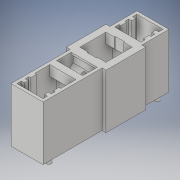
# Autodesk Inventor part: Colorimeter
Saved by Autodesk Inventor 2019 (Build 230136000, 136)
## iProperties
Created: 2019-03-27
Part Number: Colorimeter
Material: Generic
Document SubType Name: Modeling
Designer: Hansen
Density: 1 g/cm^3
Appearance: Default
Author: Hansen
Autodesk Inventor part; units mm, degrees
ref_plane "YZ Plane" through (0, 0, 0) normal (1, 0, 0) x (0, 1, 0)
ref_plane "XZ Plane" through (0, 0, 0) normal (0, 1, 0) x (-1, 0, 0)
ref_plane "XY Plane" through (0, 0, 0) normal (0, 0, 1) x (1, 0, 0)
sketch "BasePlateSketch" plane through (0, 0, 0) normal (0, 1, 0) x (-1, 0, 0)
  line L0 (-8.25, 32.5) -> (8.25, 32.5)
  line L1 (8.25, 32.5) -> (8.25, -32.5)
  line L2 (8.25, -32.5) -> (-8.25, -32.5)
  line L3 (-8.25, -32.5) -> (-8.25, 32.5)
  line L4 (-8.25, 32.5) -> (8.25, -32.5) construction
  line L5 (8.25, 32.5) -> (-8.25, -32.5) construction
  circle A0 centre (0, 28) radius 1.35
  circle A1 centre (0, -28) radius 1.35
  line L6 (-5.85, -25.25) -> (5.85, -25.25)
  line L7 (5.85, -25.25) -> (5.85, -21.75)
  line L8 (5.85, -21.75) -> (-5.85, -21.75)
  line L9 (-5.85, -21.75) -> (-5.85, -25.25)
  line L10 (-5.85, -25.25) -> (5.85, -21.75) construction
  line L11 (5.85, -25.25) -> (-5.85, -21.75) construction
  line L12 (-5.85, 25.25) -> (5.85, 25.25)
  line L13 (5.85, 25.25) -> (5.85, 21.75)
  line L14 (5.85, 21.75) -> (-5.85, 21.75)
  line L15 (-5.85, 21.75) -> (-5.85, 25.25)
  line L16 (-5.85, 25.25) -> (5.85, 21.75) construction
  line L17 (5.85, 25.25) -> (-5.85, 21.75) construction
  line L18 (4.375, 7) -> (-4.375, 7)
  line L19 (-4.375, 7) -> (-4.375, 2)
  line L20 (-4.375, 2) -> (4.375, 2)
  line L21 (4.375, 2) -> (4.375, 7)
  line L22 (4.375, 7) -> (-4.375, 2) construction
  line L23 (-4.375, 7) -> (4.375, 2) construction
  point P0 (0, 0)
  point P1 (0, 0)
  point P2 (0, 0)
  point P3 (0, -23.5)
  point P4 (0, -23.5)
  point P5 (0, 23.5)
  point P6 (0, 23.5)
  point P7 (0, 4.5)
  point P8 (0, 4.5)
  dimension "d0" = 16.5
  dimension "d1" = 65
  dimension "d2" = 4.5
  dimension "d3" = 2.7
  dimension "d4" = 4.5
  dimension "d21" = 11.7
  dimension "d22" = 3.5
  dimension "d23" = 9
  dimension "d24" = 9
  dimension "d25" = 5
  dimension "d26" = 8.75
  dimension "d27" = 25.5
  constraints: 48 end point, 13 midpoint, 8 parallel, 5 vertical alignment, 4 horizontal, 4 perpendicular, 2 centre point, 2 equal length, 1 equal radius
  measures "d0" distance of L1.end L2.end
  measures "d1" distance of L0.end L1.end
  measures "d2" distance from line of L2 A1.centre
  measures "d3" diameter of A1
  measures "d4" distance from line of L0 A0.centre
  measures "d21" distance of L6.start L6.end
  measures "d22" distance of L6.end L7.end
  measures "d23" distance from line of L2 point (0, -23.5)
  measures "d24" distance from line of point (0, 23.5) L0
  measures "d25" distance of L18.end L19.end
  measures "d26" distance of L18.start L18.end
  measures "d27" distance between parallel lines of L0 L18
extrude "BasePlate" add sketch "BasePlateSketch" along normal blind 3
sketch "SeparationsSketch" plane through (8.25, 0, 32.5) normal (1, 0, 0) x (0, 0, -1)
  line L0 (0, 3) -> (65, 3) projected
  line L1 (47.5, 3) -> (51, 3)
  line L2 (47.5, 3) -> (47.5, 5)
  line L3 (47.5, 5) -> (51, 8.5)
  line L4 (51, 8.5) -> (51, 19.25)
  line L5 (51, 19.25) -> (47.5, 22.75)
  line L6 (47.5, 22.75) -> (47.5, 28)
  line L7 (47.5, 28) -> (51, 28)
  line L8 (51, 28) -> (51, 22.75)
  line L9 (51, 22.75) -> (54.5, 19.25)
  line L10 (54.5, 19.25) -> (54.5, 8.5)
  line L11 (54.5, 8.5) -> (51, 5)
  line L12 (51, 5) -> (51, 3)
  line L13 (30.5, 3) -> (34, 3)
  line L14 (34, 3) -> (34, 13)
  line L15 (34, 13) -> (30.5, 16.5)
  line L16 (30.5, 16.5) -> (30.5, 19.25)
  line L17 (30.5, 19.25) -> (34, 22.75)
  line L18 (34, 22.75) -> (34, 28)
  line L19 (34, 28) -> (30.5, 28)
  line L20 (30.5, 28) -> (30.5, 22.75)
  line L21 (30.5, 22.75) -> (27, 19.25)
  line L22 (27, 19.25) -> (27, 16.5)
  line L23 (27, 16.5) -> (30.5, 13)
  line L24 (30.5, 13) -> (30.5, 3)
  line L25 (25.5, 0) -> (25.5, 3) projected
  line L26 (25.5, 3) -> (22, 3)
  line L27 (65, 3) -> (0, 3) projected
  line L28 (25.5, 3) -> (25.5, 19.25)
  line L29 (25.5, 19.25) -> (22, 22.75)
  line L30 (22, 22.75) -> (22, 28)
  line L31 (22, 28) -> (18.5, 28)
  line L32 (22, 3) -> (22, 19.25)
  line L33 (22, 19.25) -> (18.5, 22.75)
  line L34 (18.5, 22.75) -> (18.5, 28)
  point P0 (32.5, 0)
  point P1 (52.75, 21)
  point P2 (49.25, 21)
  point P3 (52.75, 6.75)
  point P4 (49.25, 6.75)
  point P5 (32.25, 21)
  point P6 (28.75, 21)
  point P7 (32.25, 14.75)
  point P8 (28.75, 14.75)
  point P9 (23.75, 21)
  point P10 (20.25, 21)
  dimension "d7" = 3.5
  dimension "d8" = 3.5
  dimension "d9" = 14
  dimension "d10" = 18
  dimension "d11" = 25
  dimension "d13" = 2
  dimension "d14" = 135
  dimension "d16" = 3.5
  dimension "d18" = 13.5
  dimension "d19" = 10
  dimension "d20" = 135
  dimension "d28" = 135
  constraints: 64 end point, 12 parallel, 11 point on line, 10 midpoint, 9 horizontal alignment, 8 perpendicular, 4 vertical, 3 collinear, 3 vertical alignment
  measures "d7" distance between parallel lines of L8 L6
  measures "d8" distance between parallel lines of L10 L4
  measures "d9" distance of L0.end L1.end
  measures "d10" distance from line of L1 point (52.75, 21)
  measures "d11" distance between parallel lines of L1 L7
  measures "d13" distance of L1.start L2.end
  measures "d14" angle of L4 L5
  measures "d16" distance between parallel lines of L16 L22
  measures "d18" distance between parallel lines of L6 L18
  measures "d19" distance of L13.end L14.end
  measures "d20" angle of L16 L17
  measures "d28" angle of L32 L33
extrude "Separations" add sketch "SeparationsSketch" against normal blind 16.5
sketch "Aperture1Sketch" plane through (8.25, 22.75, 14) normal (0, 0, 1) x (1, 0, 0)
  circle A0 centre (-8.25, -1.75) radius 1.5
  line L0 (-16.5, -19.75) -> (0, -19.75) projected
  line L1 (0, -22.75) -> (-16.5, -22.75) projected
  point P0 (-8.25, -22.75)
  point P1 (-8.25, -22.75)
  dimension "d31" = 3
  dimension "d32" = 18
  constraints: 1 centre point, 1 midpoint, 1 vertical alignment
  measures "d31" diameter of A0
  measures "d32" distance from line of L0 A0.centre
extrude "Aperture1" cut sketch "Aperture1Sketch" against normal up to surface (8.5 mm away)
sketch "Aperture2Sketch" plane through (8.25, 16.5, 5.5) normal (0, 0, 1) x (1, 0, 0)
  circle A0 centre (-8.25, 4.5) radius 1.5 projected
  circle A1 centre (-8.25, 4.5) radius 1.375
  point P0 (-8.25, -16.5)
  dimension "d35" = 2.75
  constraints: 1 centre point, 1 coincident
  measures "d35" diameter of A1
extrude "Aperture2" cut sketch "Aperture2Sketch" against normal up to surface (20.5 mm away) contours A1
sketch "Aperture3Sketch" plane through (8.25, 8.5, -22) normal (0, 0, -1) x (-1, 0, 0)
  circle A0 centre (8.25, 12.5) radius 1.375 projected
  circle A1 centre (8.25, 12.5) radius 1
  point P0 (8.25, -8.5)
  point P1 (7.989, 11.65)
  point P2 (7.989, 14.35)
  dimension "d38" = 2
  constraints: 1 centre point, 1 coincident, 1 other
  measures "d38" diameter of A1
extrude "Aperture3" cut sketch "Aperture3Sketch" against normal up to surface (20.5 mm away) contours A1
sketch "ApertureRefSketch" plane through (8.25, 3, 10.5) normal (0, 0, 1) x (1, 0, 0)
  line L0 (-16.5, 0) -> (0, 0) projected
  line L1 (-9.75, 7) -> (-6.75, 7)
  line L2 (-6.75, 7) -> (-6.75, 0)
  line L3 (-6.75, 0) -> (-9.75, 0)
  line L4 (-9.75, 0) -> (-9.75, 7)
  line L5 (-9.75, 7) -> (-6.75, 0) construction
  line L6 (-6.75, 7) -> (-9.75, 0) construction
  line L7 (0, -3) -> (-16.5, -3) projected
  point P0 (-8.25, -3)
  point P1 (-8.25, 3.5)
  point P2 (-8.25, 3.5)
  point P3 (-8.25, -3)
  dimension "d41" = 7
  dimension "d42" = 3
  constraints: 12 end point, 4 midpoint, 2 parallel, 1 horizontal, 1 perpendicular, 1 point on line, 1 vertical alignment
  measures "d41" distance of L3.end L1.start
  measures "d42" distance of L1.start L1.end
extrude "ApertureRef" cut sketch "ApertureRefSketch" against normal up to next
chamfer "ApertureRefChamfer" distance 3 angle 45 1 edges at (0, 10, 10.5)
sketch "OverlapSketch" plane through (8.25, 28, -15) normal (0, 1, 0) x (1, 0, 0)
  line L0 (0, 0) -> (-16.5, 0) projected
  line L1 (0, 17.5) -> (0, -47.5) projected
  line L2 (-16.5, 0) -> (0, 0)
  line L3 (0, 0) -> (0, 4.5)
  line L4 (0, 4.5) -> (-16.5, 4.5)
  line L5 (-16.5, 4.5) -> (-16.5, 0)
  line L6 (0, -13.5) -> (-16.5, -13.5) projected
  line L7 (0, -17) -> (0, -20.5) projected
  line L8 (-16.5, -13.5) -> (0, -13.5)
  line L9 (0, -13.5) -> (0, -18)
  line L10 (0, -18) -> (-16.5, -18)
  line L11 (-16.5, -18) -> (-16.5, -13.5)
  line L12 (0, -17) -> (-16.5, -17) projected
  line L13 (0, 3.5) -> (-16.5, 3.5) projected
  point P0 (-8.25, -15)
  dimension "d48" = 1
  dimension "d49" = 1
  constraints: 16 end point, 4 parallel, 2 horizontal, 2 perpendicular, 2 point on line
  measures "d48" distance between parallel lines of L10 L12
  measures "d49" distance between parallel lines of L13 L4
extrude "Overlap" add sketch "OverlapSketch" against normal blind 1
sketch "SampleProtectionCutoutSketch" plane through (-8.25, 28, -15) normal (0, 1, 0) x (1, 0, 0)
  line L0 (16.5, -13.5) -> (0, -13.5) projected
  line L1 (5.75, -13.5) -> (10.75, -13.5)
  line L2 (10.75, -13.5) -> (10.75, -14)
  line L3 (10.75, -14) -> (5.75, -14)
  line L4 (5.75, -14) -> (5.75, -13.5)
  line L5 (16.5, 0) -> (0, 0) projected
  line L6 (5.75, 0) -> (10.75, 0)
  line L7 (10.75, 0) -> (10.75, 0.5)
  line L8 (10.75, 0.5) -> (5.75, 0.5)
  line L9 (5.75, 0.5) -> (5.75, 0)
  point P0 (8.25, -15)
  point P1 (8.25, -13.5)
  point P2 (8.25, -13.5)
  dimension "d52" = 0.5
  dimension "d53" = 5
  constraints: 16 end point, 4 parallel, 4 point on line, 2 horizontal, 2 midpoint, 2 perpendicular, 1 collinear, 1 vertical alignment
  measures "d52" distance of L3.end L1.start
  measures "d53" distance of L2.end L3.end
extrude "SampleProtectionCutout" cut sketch "SampleProtectionCutoutSketch" against normal blind 25
sketch "ModuleSlidersSketch" plane through (0, 3, 0) normal (0, 1, 0) x (1, 0, 0)
  line L0 (-5.85, -25.25) -> (-5.85, -21.75) projected
  line L1 (-8.25, -32.5) -> (-8.25, 32.5) projected
  line L2 (-5.85, -21.75) -> (-8.25, -21.75)
  line L3 (-8.25, -21.75) -> (-8.25, -24.75)
  line L4 (-8.25, -24.75) -> (-5.85, -24.75)
  line L5 (-5.85, -24.75) -> (-5.85, -21.75)
  line L6 (8.25, 32.5) -> (8.25, -32.5) projected
  line L7 (5.85, -21.75) -> (8.25, -21.75)
  line L8 (8.25, -21.75) -> (8.25, -24.75)
  line L9 (8.25, -24.75) -> (5.85, -24.75)
  line L10 (5.85, -24.75) -> (5.85, -21.75)
  line L11 (-5.85, 25.25) -> (-5.85, 21.75) projected
  line L12 (-5.85, 21.75) -> (-8.25, 21.75)
  line L13 (-8.25, 21.75) -> (-8.25, 24.75)
  line L14 (-8.25, 24.75) -> (-5.85, 24.75)
  line L15 (-5.85, 24.75) -> (-5.85, 21.75)
  line L16 (-5.85, 21.75) -> (5.85, 21.75) projected
  line L17 (5.85, 21.75) -> (8.25, 21.75)
  line L18 (8.25, 21.75) -> (8.25, 24.75)
  line L19 (8.25, 24.75) -> (5.85, 24.75)
  line L20 (5.85, 24.75) -> (5.85, 21.75)
  line L21 (-8.25, -28.75) -> (-5.25, -28.75)
  line L22 (-5.25, -28.75) -> (-5.25, -26.75)
  line L23 (-5.25, -26.75) -> (-8.25, -26.75)
  line L24 (-8.25, -26.75) -> (-8.25, -28.75)
  line L25 (8.25, -28.75) -> (5.25, -28.75)
  line L26 (5.25, -28.75) -> (5.25, -26.75)
  line L27 (5.25, -26.75) -> (8.25, -26.75)
  line L28 (8.25, -26.75) -> (8.25, -28.75)
  line L29 (-8.25, 26.75) -> (-5.25, 26.75)
  line L30 (-5.25, 26.75) -> (-5.25, 28.75)
  line L31 (-5.25, 28.75) -> (-8.25, 28.75)
  line L32 (-8.25, 28.75) -> (-8.25, 26.75)
  line L33 (8.25, 28.75) -> (5.25, 28.75)
  line L34 (5.25, 28.75) -> (5.25, 26.75)
  line L35 (5.25, 26.75) -> (8.25, 26.75)
  line L36 (8.25, 26.75) -> (8.25, 28.75)
  line L37 (-8.25, -32.5) -> (8.25, -32.5) projected
  line L38 (8.25, 32.5) -> (-8.25, 32.5) projected
  point P0 (0, 0)
  dimension "d56" = 2
  dimension "d57" = 2
  dimension "d58" = 2
  dimension "d59" = 10.5
  dimension "d60" = 3.75
  dimension "d61" = 3.75
  constraints: 64 end point, 16 parallel, 16 point on line, 8 horizontal, 8 perpendicular, 2 collinear
  measures "d56" distance between parallel lines of L4 L23
  measures "d57" distance between parallel lines of L29 L14
  measures "d58" distance of L21.end L22.end
  measures "d59" distance between parallel lines of L26 L22
  measures "d60" distance between parallel lines of L37 L21
  measures "d61" distance between parallel lines of L38 L31
extrude "ModuleSliders" add sketch "ModuleSlidersSketch" along normal blind 25 contours L4 L1 L2 L0 | L23 L22 L21 L1 | L1 L14 L11 L12 | L1 L31 L30 L29 | L20 L19 L6 L17 | L25 L26 L27 L6 | L6 L9 L10 L7 | L35 L34 L33 L6
sketch "BaseplateComponentsCutoutSketch" plane through (0, 0, 0) normal (0, -1, 0) x (1, 0, 0)
  line L0 (-4.375, 7) -> (4.375, 7) projected
  line L1 (3, 7) -> (-3, 7)
  line L2 (-3, 7) -> (-3, 9)
  line L3 (-3, 9) -> (3, 9)
  line L4 (3, 9) -> (3, 7)
  line L5 (5.25, 20) -> (-5.25, 20)
  line L6 (-5.25, 20) -> (-5.25, 15.5)
  line L7 (-5.25, 15.5) -> (5.25, 15.5)
  line L8 (5.25, 15.5) -> (5.25, 20)
  line L9 (5.85, 21.75) -> (-5.85, 21.75) projected
  point P0 (0, 0)
  point P1 (0, 9)
  point P2 (0, 15.5)
  dimension "d64" = 1.75
  dimension "d65" = 4.5
  dimension "d66" = 10.5
  dimension "d67" = 6
  dimension "d68" = 2
  constraints: 16 end point, 4 parallel, 2 horizontal, 2 midpoint, 2 perpendicular, 2 vertical alignment, 1 point on line
  measures "d64" distance between parallel lines of L5 L9
  measures "d65" distance of L7.end L5.start
  measures "d66" distance of L6.end L7.end
  measures "d67" distance of L2.end L3.end
  measures "d68" distance of L3.end L1.start
extrude "BaseplateComponentsCutout" cut sketch "BaseplateComponentsCutoutSketch" against normal blind 1
sketch "OuterWallsSketch" plane through (0, 0, 0) normal (0, -1, 0) x (1, 0, 0)
  line L0 (8.25, 32.5) -> (-8.25, 32.5) projected
  line L1 (8.25, -32.5) -> (8.25, 32.5) projected
  line L2 (-8.25, 32.5) -> (8.25, 32.5)
  line L3 (8.25, 32.5) -> (8.25, -32.5)
  line L4 (8.25, -32.5) -> (-8.25, -32.5)
  line L5 (-8.25, -32.5) -> (-8.25, 32.5)
  line L6 (6.75, 31) -> (-6.75, 31)
  line L7 (-6.75, 31) -> (-6.75, -31)
  line L8 (-6.75, -31) -> (6.75, -31)
  line L9 (6.75, -31) -> (6.75, 31)
  line L10 (8.25, 2) -> (10.25, 2)
  line L11 (10.25, 2) -> (10.25, -18.5)
  line L12 (10.25, -18.5) -> (8.25, -18.5)
  line L13 (8.25, -18.5) -> (8.25, 2)
  line L14 (-8.25, 2) -> (-10.25, 2)
  line L15 (-10.25, 2) -> (-10.25, -18.5)
  line L16 (-10.25, -18.5) -> (-8.25, -18.5)
  line L17 (-8.25, -18.5) -> (-8.25, 2)
  point P0 (0, 0)
  point P1 (6.75, 0)
  point P2 (0, -31)
  dimension "d72" = 13.5
  dimension "d73" = 1.5
  dimension "d74" = 3.5
  constraints: 32 end point, 8 parallel, 4 horizontal, 4 perpendicular, 4 point on line, 2 coincident, 2 midpoint, 1 collinear, 1 horizontal alignment, 1 vertical alignment
  measures "d72" distance between parallel lines of L7 L9
  measures "d73" distance between parallel lines of L4 L8
  measures "d74" distance between parallel lines of L9 L11
extrude "OuterWalls" add sketch "OuterWallsSketch" against normal blind 28
sketch "ExpansionHeaderCutoutSketch" plane through (0, 0, 0) normal (0, -1, 0) x (1, 0, 0)
  line L0 (-10.25, -18.5) -> (-10.25, 2) projected
  line L1 (-10.25, -6) -> (-6.5, -6)
  line L2 (-6.5, -6) -> (-6.5, -19)
  line L3 (-6.5, -19) -> (-10.25, -19)
  line L4 (-10.25, -19) -> (-10.25, -6)
  line L5 (-8.25, -32.5) -> (8.25, -32.5) projected
  point P0 (0, 0)
  dimension "d77" = 13.5
  dimension "d78" = 13
  dimension "d82" = 3.75
  constraints: 8 end point, 2 parallel, 1 horizontal, 1 perpendicular, 1 point on line
  measures "d77" distance between parallel lines of L5 L3
  measures "d78" distance between parallel lines of L3 L1
  measures "d82" distance of L1.start L1.end
extrude "ExpansionHeaderCutout" cut sketch "ExpansionHeaderCutoutSketch" against normal blind 2
sketch "AlignmentPadsSketch" plane through (0, 0, 0) normal (0, -1, 0) x (1, 0, 0)
  circle A0 centre (6.75, 28) radius 1.25
  circle A1 centre (6.75, -28) radius 1.25
  circle A2 centre (-6.75, -28) radius 1.25
  circle A3 centre (-6.75, 28) radius 1.25
  line L0 (8.25, -32.5) -> (8.25, -18.5) projected
  line L1 (-8.25, -32.5) -> (8.25, -32.5) projected
  point P0 (0, 0)
  dimension "d83" = 2.5
  dimension "d84" = 56
  dimension "d85" = 13.5
  dimension "d86" = 1.5
  dimension "d87" = 4.5
  constraints: 4 centre point, 3 equal radius, 2 horizontal alignment, 2 vertical alignment
  measures "d83" diameter of A0
  measures "d84" distance of A1.centre A0.centre
  measures "d85" distance of A3.centre A0.centre
  measures "d86" distance from line of A1.centre L0
  measures "d87" distance from line of L1 A1.centre
extrude "Extrusion13" add sketch "AlignmentPadsSketch" along normal blind 2
equation "\"d4\" = d2"
equation "\"d24\" = d23"
equation "\"d8\" = d7"
equation "\"d16\" = d7"
equation "\"d20\" = d14"
equation "\"d28\" = d14"
equation "\"d29\" = d0"
equation "\"d32\" = d10"
equation "\"d49\" = d48"
equation "\"d54\" = d11"
equation "\"d57\" = d56"
equation "\"d61\" = d60"
equation "\"d62\" = d11"
equation "\"d72\" = d18"
equation "\"d74\" = d7"
equation "\"d75\" = d5 + d11"
equation "\"d5\" = 3"
body "Solid1"
